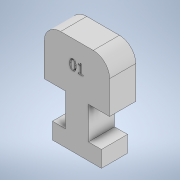
# Autodesk Inventor part: 01_02
Saved by Autodesk Inventor 2021 (Build 250183000, 183)
## iProperties
Created: 2025-03-19
Part Number: 01_02
Material: 일반
Document SubType Name: Modeling
Designer: USER
Density: 1 g/cm^3
Appearance: 기본값
Author: USER
Autodesk Inventor part; units mm, degrees
ref_plane "YZ Plane" through (0, 0, 0) normal (1, 0, 0) x (0, 1, 0)
ref_plane "XZ Plane" through (0, 0, 0) normal (0, 1, 0) x (-1, 0, 0)
ref_plane "XY Plane" through (0, 0, 0) normal (0, 0, 1) x (1, 0, 0)
sketch "스케치1" plane through (0, 0, 0) normal (0, 0, 1) x (1, 0, 0)
  line L0 (-5, 14) -> (5, 14)
  line L1 (7.5, -16.0251) -> (-7.5, -16.0251)
  line L2 (-7.5, -11.0251) -> (-7.5, -16.0251)
  line L3 (3.5, -1.0251) -> (3.5, -11.0251)
  line L4 (-3.5, -11.0251) -> (-3.5, -1.0251)
  line L5 (7.5, -11.0251) -> (7.5, -16.0251)
  line L6 (-3.5, -1.0251) -> (-10, -1.0251)
  line L7 (-3.5, -1.0251) -> (3, -1.0251) construction
  line L8 (3.5, -1.0251) -> (10, -1.0251)
  line L9 (3.5, -1.0251) -> (10, -1.0251) construction
  line L10 (-10, 9) -> (-10, -1.0251)
  line L11 (10, -1.0251) -> (10, 9)
  line L12 (-7.5, -11.0251) -> (-3.5, -11.0251)
  line L13 (3.5, -11.0251) -> (7.5, -11.0251)
  arc A0 (-5, 14) -> (-10, 9) centre (-5, 9) ccw
  arc A1 (10, 9) -> (5, 14) centre (5, 9) ccw
  point P0 (0, 0)
  point P1 (-10, 14)
  point P2 (10, 14)
  dimension "d2" = 20
  dimension "d5" = 15
  dimension "d7" = 7.5
  dimension "d12" = 7
  dimension "d13" = 3.5
  dimension "d14" = 180
  dimension "d15" = 0
  dimension "d16" = 5
  dimension "d17" = 5
  dimension "d18" = 10
  constraints: 29 end point, 5 horizontal, 4 point on circle, 4 point on line, 4 tangent, 2 centre point, 2 collinear, 2 perpendicular, 2 vertical, 1 equal radius, 1 parallel
  measures "d2" distance of point (-10, 14) point (10, 14)
  measures "d5" distance of L2.start L5.start
  measures "d7" distance from line of L2 point (0, 0)
  measures "d12" distance of L3.end L4.start
  measures "d13" distance from line of L3 point (0, 0)
  measures "d14" angle of L6 L7
  measures "d15" distance between parallel lines of L8 L9
  measures "d16" radius of A0
  measures "d17" distance of L5.start L1.start
  measures "d18" distance of L3.start L3.end
sketch "스케치2" plane through (0, 0, 0) normal (0, 0, 1) x (1, 0, 0)
  line L0 (10, -1) -> (3.4836, -1)
  point P0 (0, 0)
  constraints: 2 end point, 1 horizontal
sketch "스케치3" plane through (0, 0, 0) normal (0, 0, 1) x (1, 0, 0)
  point P0 (0, 0)
extrude "돌출1" add sketch "스케치1" along normal blind 8
sketch "스케치4" plane through (0, 0, 8) normal (0, 0, 1) x (1, 0, 0)
  line L0 (-2.3546, 8.6646) -> (2.2199, 8.6646) construction
  line L1 (2.2199, 8.6646) -> (2.2199, 5.4907) construction
  line L2 (2.2199, 5.4907) -> (-2.3546, 5.4907) construction
  line L3 (-2.3546, 5.4907) -> (-2.3546, 8.6646) construction
  spline S0 degree 2 poles (-0.2353, 7.0789) (-0.2353, 6.2588) (-0.712, 5.4907) (-1.2085, 5.4907) knots 0 0 0 1 2 2 2
  spline S1 degree 2 poles (-1.2085, 5.4907) (-1.7124, 5.4907) (-2.1841, 6.2737) (-2.1841, 7.0764) knots 0 0 0 1 2 2 2
  spline S2 degree 2 poles (-2.1841, 7.0764) (-2.1841, 7.9014) (-1.7074, 8.6646) (-1.2085, 8.6646) knots 0 0 0 1 2 2 2
  spline S3 degree 2 poles (-1.2085, 8.6646) (-0.7071, 8.6646) (-0.2353, 7.8742) (-0.2353, 7.0789) knots 0 0 0 1 2 2 2
  spline S4 degree 2 poles (-0.7589, 6.1502) (-0.6997, 6.3008) (-0.6503, 6.7652) (-0.6503, 7.0789) knots 0 0 0 1 2 2 2
  spline S5 degree 2 poles (-0.6503, 7.0789) (-0.6503, 7.3926) (-0.6997, 7.8545) (-0.7614, 8.0101) knots 0 0 0 1 2 2 2
  spline S6 degree 2 poles (-0.7614, 8.0101) (-0.8232, 8.1657) (-1.0381, 8.3263) (-1.2085, 8.3263) knots 0 0 0 1 2 2 2
  spline S7 degree 2 poles (-1.2085, 8.3263) (-1.3789, 8.3263) (-1.5988, 8.1657) (-1.663, 8.0052) knots 0 0 0 1 2 2 2
  spline S8 degree 2 poles (-1.663, 8.0052) (-1.7247, 7.8495) (-1.7692, 7.3753) (-1.7692, 7.0764) knots 0 0 0 1 2 2 2
  spline S9 degree 2 poles (-1.7692, 7.0764) (-1.7692, 6.7553) (-1.7297, 6.3255) (-1.6654, 6.1576) knots 0 0 0 1 2 2 2
  spline S10 degree 2 poles (-1.6654, 6.1576) (-1.6062, 5.9995) (-1.3863, 5.8291) (-1.2085, 5.8291) knots 0 0 0 1 2 2 2
  spline S11 degree 2 poles (-1.2085, 5.8291) (-1.0405, 5.8291) (-0.8207, 5.9896) (-0.7589, 6.1502) knots 0 0 0 1 2 2 2
  line L4 (1.8815, 5.5549) -> (0.3945, 5.5549)
  line L5 (0.3945, 5.5549) -> (0.3945, 5.8661)
  line L6 (0.3945, 5.8661) -> (0.9478, 5.8661)
  line L7 (0.9478, 5.8661) -> (0.9478, 7.9088)
  line L8 (0.9478, 7.9088) -> (0.3945, 7.9088)
  line L9 (0.3945, 7.9088) -> (0.3945, 8.1879)
  spline S12 degree 2 poles (0.3945, 8.1879) (0.7082, 8.1879) (1.0046, 8.3658) (1.0244, 8.6128) knots 0 0 0 1 2 2 2
  line L10 (1.0244, 8.6128) -> (1.3406, 8.6128)
  line L11 (1.3406, 8.6128) -> (1.3406, 5.8661)
  line L12 (1.3406, 5.8661) -> (1.8815, 5.8661)
  line L13 (1.8815, 5.8661) -> (1.8815, 5.5549)
  point P0 (0, 0)
  constraints: 2 other
extrude "돌출2" cut sketch "스케치4" against normal blind 3
